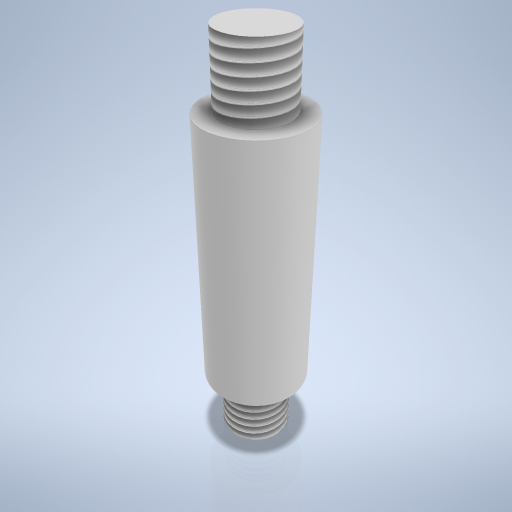
# Autodesk Inventor part: 8
Saved by Autodesk Inventor 2024.2 (Build 282272000, 272)
## iProperties
Created: 2024-05-04
Part Number: 8
Material: Generisch
Document SubType Name: Modeling
Designer: Fabri
Density: 1 g/cm^3
Appearance: Vorgabe
Author: Fabri
Autodesk Inventor part; units mm, degrees
ref_plane "YZ Plane" through (0, 0, 0) normal (1, 0, 0) x (0, 1, 0)
ref_plane "XZ Plane" through (0, 0, 0) normal (0, 1, 0) x (-1, 0, 0)
ref_plane "XY Plane" through (0, 0, 0) normal (0, 0, 1) x (1, 0, 0)
sketch "Skizze1" plane through (0, 0, 0) normal (0, 1, 0) x (-1, 0, 0)
  line L0 (0, 30) -> (5, 30)
  line L1 (5, 30) -> (5, 20)
  line L2 (5, 20) -> (7.5, 20)
  line L3 (7.5, 20) -> (7.5, -20)
  line L4 (7.5, -20) -> (5, -20)
  line L5 (5, -20) -> (5, -30)
  line L6 (5, -30) -> (0, -30)
  line L7 (0, -30) -> (0, 30)
  line L8 (0, 0) -> (12.831, 0) construction
  dimension "d0" = 10
  dimension "d1" = 10
  dimension "d2" = 40
  dimension "d3" = 10
  dimension "d4" = 15
  constraints: 18 end point, 6 perpendicular, 2 horizontal, 2 point on line, 1 coincident, 1 midpoint
  measures "d0" distance of L0.end L1.end
  measures "d1" distance between parallel lines of L6 L4
  measures "d2" distance of L2.end L3.end
  measures "d3" diameter of L1 L7
  measures "d4" diameter of L3 L7
revolve "Umdrehung1" add sketch "Skizze1" angle 360 about axis through (0, 0, -30) along (0, 0, 1)
thread "Gewinde1" size "M10x1.5" class "6g" standard "ISO Metric profile" full length
